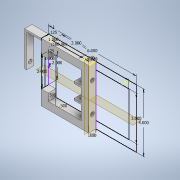
# Autodesk Inventor part: SampleHolder
Saved by Autodesk Inventor 2020 (Build 240168000, 168)
## iProperties
Created: 2022-01-27
Part Number: SampleHolder
Material: Generic
Document SubType Name: Modeling
Designer: Beaucage
Density: 1 g/cm^3
Appearance: Default
Author: Beaucage
Autodesk Inventor part; units mm, degrees
ref_plane "YZ Plane" through (0, 0, 0) normal (1, 0, 0) x (0, 1, 0)
ref_plane "XZ Plane" through (0, 0, 0) normal (0, 1, 0) x (-1, 0, 0)
ref_plane "XY Plane" through (0, 0, 0) normal (0, 0, 1) x (1, 0, 0)
sketch "Sketch1" plane through (0, 0, 0) normal (0, 0, 1) x (1, 0, 0)
  line L0 (0, 0) -> (152.4, 0)
  line L1 (152.4, 0) -> (152.4, 101.6)
  line L2 (152.4, 101.6) -> (0, 101.6)
  line L3 (0, 101.6) -> (0, 0)
  line L4 (0, 0) -> (12.7, 0)
  line L5 (12.7, 0) -> (12.7, 12.7)
  line L6 (12.7, 12.7) -> (139.7, 12.7)
  line L7 (139.7, 12.7) -> (139.7, 88.9)
  line L8 (139.7, 88.9) -> (12.7, 88.9)
  line L9 (12.7, 88.9) -> (12.7, 12.7)
  line L10 (69.85, 101.6) -> (82.55, 101.6)
  line L11 (82.55, 101.6) -> (82.55, 0)
  line L12 (82.55, 0) -> (69.85, 0)
  line L13 (69.85, 0) -> (69.85, 101.6)
  line L14 (69.85, 101.6) -> (82.55, 0) construction
  line L15 (82.55, 101.6) -> (69.85, 0) construction
  point P0 (76.2, 50.8)
  point P1 (82.55, 88.9)
  point P2 (82.55, 12.7)
  point P3 (69.85, 12.7)
  point P4 (69.85, 88.9)
  dimension "d0" = 152.4
  dimension "d1" = 101.6
  dimension "d2" = 12.7
  dimension "d3" = 12.7
  dimension "d4" = 127
  dimension "d5" = 76.2
  dimension "d6" = 12.7
  constraints: 32 end point, 6 parallel, 4 perpendicular, 3 horizontal, 2 midpoint, 2 point on line
  measures "d0" distance of L2.end L1.end
  measures "d1" distance of L1.end L0.end
  measures "d2" distance of L0.start L4.end
  measures "d3" distance of L4.end L5.end
  measures "d4" distance of L8.end L7.end
  measures "d5" distance of L7.end L6.end
  measures "d6" distance of L11.end L12.end
extrude "Extrusion1" add sketch "Sketch1" along normal blind 12.7 contours L3 L2 L13 L8 L9 L5 L0 | L5 L6 L13 L0 | L13 L6 L11 L0 | L2 L11 L8 L13 | L11 L6 L7 L8 L2 L1 L0 | L13 L8 L11 L6
sketch "Sketch2" plane through (0, 101.6, 0) normal (0, 1, 0) x (1, 0, 0)
  line L0 (69.85, 0) -> (69.85, -12.7) projected
  line L1 (82.55, 0) -> (82.55, -12.7) projected
  line L2 (139.7, 0) -> (139.7, -12.7) projected
  line L3 (12.7, 0) -> (12.7, -12.7) projected
  line L4 (12.7, 0) -> (12.7, -12.7) projected
  line L5 (12.7, -6.35) -> (63.5, -6.35)
  line L6 (69.85, -6.35) -> (76.2, -6.35)
  point P0 (0, 0)
  dimension "d9" = 50.8
  dimension "d17" = 6.35
  constraints: 4 end point, 2 midpoint, 2 perpendicular, 1 coincident
  measures "d9" distance of L5.start L5.end
  measures "d17" distance of L6.start L6.end
sketch "Sketch4" plane through (69.85, 12.7, 0) normal (1, 0, 0) x (0, 0, -1)
  line L0 (0, 76.2) -> (-12.7, 76.2) projected
  line L1 (-6.35, 76.2) -> (-6.35, 50.8)
  line L2 (-6.35, 76.2) -> (19.05, 76.2) construction
  line L3 (-6.35, 50.8) -> (-6.35, 25.4)
  line L4 (0, 0) -> (0, 76.2) projected
  line L5 (-12.7, 52.3875) -> (0, 52.3875)
  line L6 (0, 52.3875) -> (0, 49.2125)
  line L7 (0, 49.2125) -> (-12.7, 49.2125)
  line L8 (-12.7, 49.2125) -> (-12.7, 52.3875)
  line L9 (-12.7, 52.3875) -> (0, 49.2125) construction
  line L10 (0, 52.3875) -> (-12.7, 49.2125) construction
  line L11 (-12.7, 23.8125) -> (0, 23.8125)
  line L12 (0, 23.8125) -> (0, 26.9875)
  line L13 (0, 26.9875) -> (-12.7, 26.9875)
  line L14 (-12.7, 26.9875) -> (-12.7, 23.8125)
  line L15 (-12.7, 23.8125) -> (0, 26.9875) construction
  line L16 (0, 23.8125) -> (-12.7, 26.9875) construction
  point P0 (0, -12.7)
  dimension "d25" = 25.4
  dimension "d26" = 90
  dimension "d27" = 25.4
  dimension "d28" = 180
  dimension "d29" = 3.175
  dimension "d30" = 3.175
  constraints: 30 end point, 5 equal length, 5 midpoint, 3 horizontal, 3 perpendicular, 2 point on line, 1 vertical
  measures "d25" distance of L1.start L1.end
  measures "d26" angle of L1 L2
  measures "d27" distance of L1.end L3.end
  measures "d28" angle of L3 L1
  measures "d29" distance of L5.end L6.end
  measures "d30" distance of L12.end L11.end
extrude "Extrusion2" add sketch "Sketch4" against normal blind 12.7 contours L4 L7 L3 L1 L5 | L1 L3 L7 L8 L5 | L4 L11 L14 L13
hole "Hole1" at (63.5, 101.6, 6.35) direction (0, -1, 0) diameter 1.8415 end through all both
hole "Hole2" at (63.5, 101.6, 6.35) direction (0, -1, 0) diameter 3.429 depth 3.175
ref_plane "Work Plane1" through (76.2, 101.6, 6.35) normal (1, 0, 0) x (0, 0, -1)
ref_plane "Work Plane2" through (76.2, 50.8, 0) normal (0, 1, 0) x (1, 0, 0)
mirror "Mirror1" about plane through (76.2, 101.6, 6.35) normal (1, 0, 0) of "Hole1", "Hole2", "Extrusion2"
mirror "Mirror2" about plane through (76.2, 50.8, 0) normal (0, 1, 0) of "Hole1", "Hole2", "Mirror1"
sketch "Sketch5" plane through (0, 0, 0) normal (-1, 0, 0) x (0, 0, 1)
  line L0 (12.7, 61.9125) -> (12.7, 39.6875) projected
  line L1 (12.7, 50.8) -> (12.7, 76.2)
  line L2 (12.7, 76.2) -> (0, 76.2)
  line L3 (0, 76.2) -> (0, 25.4)
  line L4 (0, 25.4) -> (12.7, 25.4)
  line L5 (12.7, 25.4) -> (12.7, 76.2)
  line L6 (4.6355, 101.6) -> (8.0645, 101.6) projected
  line L7 (6.35, 101.6) -> (6.35, 76.2)
  line L8 (6.35, 76.2) -> (6.35, 25.4)
  line L9 (0, 12.7) -> (12.7, 12.7) projected
  line L10 (0, 88.9) -> (0, 12.7) projected
  line L11 (12.7, 76.2) -> (0, 76.2)
  line L12 (0, 76.2) -> (0, 79.375)
  line L13 (0, 79.375) -> (12.7, 79.375)
  line L14 (12.7, 79.375) -> (12.7, 76.2)
  line L15 (0, 101.6) -> (12.7, 101.6) projected
  line L16 (0, 101.6) -> (0, 0) projected
  line L17 (12.7, 101.6) -> (0, 101.6)
  line L18 (0, 101.6) -> (0, 98.425)
  line L19 (0, 98.425) -> (12.7, 98.425)
  line L20 (12.7, 98.425) -> (12.7, 101.6)
  dimension "d33" = 25.4
  dimension "d34" = 50.8
  dimension "d35" = 25.4
  dimension "d36" = 50.8
  dimension "d37" = 180
  dimension "d45" = 3.175
  dimension "d62" = 3.175
  constraints: 30 end point, 6 parallel, 4 perpendicular, 3 horizontal, 2 midpoint, 1 collinear, 1 point on line, 1 vertical, 2 other
  measures "d33" distance of L1.start L1.end
  measures "d34" distance of L3.end L2.end
  measures "d35" distance of L7.start L7.end
  measures "d36" distance of L7.end L8.end
  measures "d37" angle of L8 L7
  measures "d45" distance of L11.end L12.end
  measures "d62" distance of L18.end L17.end
hole "Hole3" [suppressed]
extrude "Extrusion3" cut sketch "Sketch5" against normal blind 12.7 contours L0 L5 L4 L8 L2 L1 | L8 L4 L3 L2
extrude "Extrusion4" add sketch "Sketch5" along normal blind 28.575 contours L19 L16 L15 L6 L7 | L7 L6 L15 L20 L19
sketch "Sketch6" plane through (12.7, 98.425, 0) normal (0, -1, 0) x (1, 0, 0)
  line L0 (-12.7, 12.7) -> (0, 12.7) projected
  line L1 (0, 0) -> (-12.7, 0) projected
  line L2 (-41.275, 12.7) -> (-38.1, 12.7)
  line L3 (-38.1, 12.7) -> (-38.1, 0)
  line L4 (-38.1, 0) -> (-41.275, 0)
  line L5 (-41.275, 0) -> (-41.275, 12.7)
  dimension "d50" = 3.175
  constraints: 8 end point, 2 parallel, 1 horizontal, 1 perpendicular, 1 point on line
  measures "d50" distance of L3.end L4.end
extrude "Extrusion5" add sketch "Sketch6" along normal blind 57.15
sketch "Sketch7" plane through (-28.575, 0, 0) normal (-1, 0, 0) x (0, 0, 1)
  line L0 (12.7, 88.9) -> (12.7, 12.7) projected
  line L1 (12.7, 38.0513) -> (6.35, 38.0513)
  line L2 (5.4292, 36.5125) -> (5.4292, 39.6875) projected
  line L3 (6.35, 38.0513) -> (6.35, 50.7513)
  point P0 (0, 0)
  dimension "d53" = 6.35
  dimension "d54" = 12.7
  constraints: 4 end point, 2 perpendicular, 1 point on line
  measures "d53" distance of L1.start L1.end
  measures "d54" distance of L1.end L3.end
hole "Hole4" at (-28.575, 50.7513, 6.35) direction (1, 0, 0) diameter 6.7564 depth 25.4 clearance for "Flat Head Machine Screw (82)" size "1/4" standard "Ansi Unified Screw Threads"
mirror "Mirror3" about plane through (76.2, 101.6, 6.35) normal (1, 0, 0) of "Extrusion3", "Extrusion4", "Extrusion5", "Hole4"
sketch "Sketch8" plane through (69.85, 88.9, 0) normal (-1, 0, 0) x (0, 0, 1)
  line L0 (12.7, 0) -> (12.7, -23.8125) projected
  line L1 (12.7, 0) -> (6.35, 0)
  line L2 (12.7, 0) -> (19.05, 0) construction
  line L3 (6.35, 0) -> (6.35, -12.7)
  point P0 (0, -88.9)
  dimension "d63" = 6.35
  dimension "d64" = 180
  dimension "d65" = 12.7
  constraints: 6 end point, 2 horizontal, 1 collinear, 1 perpendicular
  measures "d63" distance of L0.start L1.end
  measures "d64" angle of L1 L2
  measures "d65" distance of L1.end L3.end
hole "Hole5" at (69.85, 76.2, 6.35) direction (1, 0, 0) diameter 6.7564 depth 25.4 counterbore diameter 11.1252 counterbore depth 6.35 clearance for "Socket Head Cap Screw" size "1/4" standard "Ansi Unified Screw Threads"
ref_plane "Work Plane3" through (82.55, 101.6, 6.35) normal (1, 0, 0) x (0, 0, -1)
split "Split1" plane through (82.55, 101.6, 6.35) removes the side toward (1, 0, 0)
mirror "Mirror4" about plane through (76.2, 50.8, 0) normal (0, 1, 0) of "Hole5"
body "Solid1"
